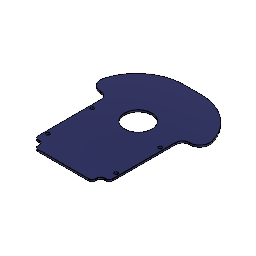
board v7 (Autodesk Fusion 360 design; units mm, degrees)
Autodesk Fusion 360 part; units mm, degrees
sketch "スケッチ1" plane through (0, 0, 0) normal (0, 0, 1) x (1, 0, 0)
  line L0 (0, 0) -> (-11, 0)
  line L1 (-11, 0) -> (-11, 12)
  line L2 (-11, 12) -> (0, 12)
  line L3 (0, 12) -> (0, 0)
  line L4 (0, 0) -> (11, 0)
  line L5 (11, 0) -> (11, 12)
  line L6 (11, 12) -> (0, 12)
  line L7 (0, 12) -> (0, 0)
  line L8 (0, 0) -> (-11, 0)
  line L9 (-11, 0) -> (-11, -9.5)
  line L10 (-11, -9.5) -> (0, -9.5)
  line L11 (0, -9.5) -> (0, 0)
  line L12 (0, 0) -> (11, 0)
  line L13 (11, 0) -> (11, -9.5)
  line L14 (11, -9.5) -> (0, -9.5)
  line L15 (0, -9.5) -> (0, 0)
  line L16 (0, -9.5) -> (-8.5, -9.5)
  line L17 (-8.5, -9.5) -> (-8.5, -12)
  line L18 (-8.5, -12) -> (0, -12)
  line L19 (0, -12) -> (0, -9.5)
  line L20 (0, -9.5) -> (8.5, -9.5)
  line L21 (8.5, -9.5) -> (8.5, -12)
  line L22 (8.5, -12) -> (0, -12)
  line L23 (0, -12) -> (0, -9.5)
  line L24 (-11, 12) -> (-16.5, 12)
  line L25 (11, 12) -> (16.5, 12)
  arc A0 (-2.5, 26) -> (-16.5, 12) centre (-2.5, 12) ccw
  arc A1 (16.5, 12) -> (2.5, 26) centre (2.5, 12) ccw
  line L26 (-2.5, 26) -> (2.5, 26)
  circle A2 centre (-10, 6.5) radius 0.5
  circle A3 centre (-10, -6.5) radius 0.5
  circle A4 centre (10, -6.5) radius 0.5
  circle A5 centre (10, 6.5) radius 0.5
  line L27 (0, 12) -> (0, 26)
  circle A6 centre (0, 10) radius 4
  dimension "d1" = 5.5
  dimension "d2" = 11
  dimension "d3" = 12
  dimension "d4" = 26
  dimension "d5" = 1
  dimension "d6" = 6.5
  dimension "d7" = 3
  dimension "d8" = 2.5
  dimension "d9" = 2.5
  dimension "d18" = 1
  dimension "d19" = 10
  dimension "d21" = 8
  measures "d4" distance of L12 L26
  measures "d5" diameter of A2
  measures "d6" distance of L0
  measures "d7" distance of L10
  measures "d18" distance of L9
  measures "d19" distance of L4
  measures "d21" diameter of A6
extrude "押し出し1" add sketch "スケッチ1" along normal blind 0.6 contours L0 L8 L9 L10 L11 L15 L16 | L0 L1 L2 L3 L7 L8 A6 | L3 L4 L5 L6 L7 L12 A6 | L4 L11 L12 L13 L14 L15 L20 | L10 L16 L17 L18 L19 L23 | L14 L19 L20 L21 L22 L23 | L2 L24 A0 L26 L27 A6 | L6 L25 A1 L26 L27 A6
fillet "フィレット1" radius 3 2 edges at (-16.5, 12, 0.3) (16.5, 12, 0.3)
fillet "フィレット1" radius 2 2 edges at (-11, 12, 0.3) (11, 12, 0.3)
fillet "フィレット1" radius 1 6 edges at (-11, -9.5, 0.3) (-8.5, -9.5, 0.3) (-8.5, -12, 0.3) (8.5, -12, 0.3) (8.5, -9.5, 0.3) (11, -9.5, 0.3)
